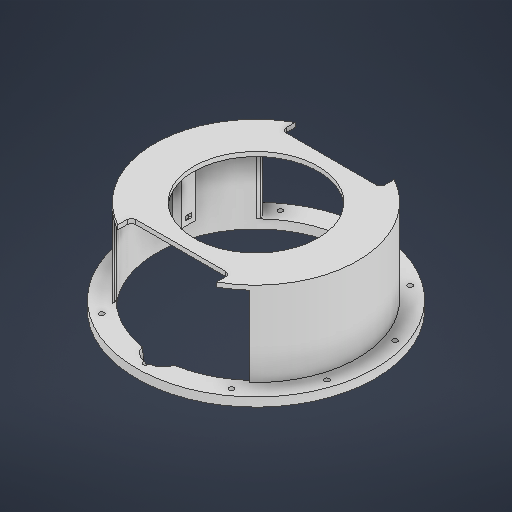
# Autodesk Inventor part: Cylinder Segment  Camera only
Saved by Autodesk Inventor 2026 (Build 300175000, 175)
## iProperties
Created: 2024-04-11
Part Number: Cylinder Segment  Camera only
Material: Generic
Document SubType Name: Modeling
Designer: Thienan Hoang
Density: 1 g/cm^3
Appearance: Default
Author: Thienan Hoang
Autodesk Inventor part; units mm, degrees
sketch "Sketch1" plane through (0, 0, 0) normal (0, 1, 0) x (-1, 0, 0)
  circle A0 centre (0, 0) radius 135
  circle A1 centre (0, 0) radius 115
  circle A2 centre (0, 0) radius 112.0375
  circle A3 centre (0, 0) radius 9.5
  circle A4 centre (0, 0) radius 125
  circle A5 centre (0, -125) radius 2.75
  circle A6 centre (73.4732, -101.1271) radius 2.75
  circle A7 centre (118.8821, -38.6271) radius 2.75
  circle A8 centre (118.8821, 38.6271) radius 2.75
  circle A9 centre (73.4732, 101.1271) radius 2.75
  circle A10 centre (0, 125) radius 2.75
  circle A11 centre (-73.4732, 101.1271) radius 2.75
  circle A12 centre (-118.8821, 38.6271) radius 2.75
  circle A13 centre (-118.8821, -38.6271) radius 2.75
  circle A14 centre (-73.4732, -101.1271) radius 2.75
  point P0 (0, -115)
  point P1 (0, -112.0375)
  point P2 (0, -135)
  point P3 (0, -112.0375)
  point P4 (0, -115)
  point P5 (0, -135)
  point P6 (0, 112.0375)
  point P7 (0, 115)
  point P8 (0, 135)
  dimension "d264" = 250
  dimension "Absolute_Diameter" = 270
  dimension "Diameter_No_Outer_Lip" = 230
  dimension "Inner_Cylinder_Diameter" = 224.075
  dimension "Lip_Diameter" = 19
  dimension "d265" = 5.5
  dimension "d268" = 360
  constraints: 14 centre point, 8 coincident, 6 point on circle, 1 vertical alignment, 23 other
  measures "Absolute_Diameter" diameter of A0
  measures "Diameter_No_Outer_Lip" diameter of A1
  measures "Inner_Cylinder_Diameter" diameter of A2
  measures "Lip_Diameter" diameter of A3
  measures "d265" diameter of A5
extrude "Extrusion1" add sketch "Sketch1" along normal blind 10 contours A0 | A4 A7 A6 A5 A14 A13 A12 A11 A10 A9 A8
extrude "Extrusion2" add sketch "Sketch1" along normal blind 105.5 contours A1
sketch "Sketch2" plane through (0, 105.5, 0) normal (0, 1, 0) x (1, 0, 0)
  circle A0 centre (0, 0) radius 115
  circle A1 centre (0, 0) radius 70.375
  dimension "Lip_Diameter_Out" = 230
  dimension "Inner_Lip_Diameter" = 140.75
  constraints: 2 centre point, 1 coincident
  measures "Lip_Diameter_Out" diameter of A0
  measures "Inner_Lip_Diameter" diameter of A1
extrude "Extrusion7" add sketch "Sketch2" against normal blind 5
sketch "Sketch28" plane through (0, 10, 0) normal (0, 1, 0) x (1, 0, 0)
  line L0 (-77.5, -75) -> (77.5, -75)
  line L1 (77.5, -75) -> (77.5, -175)
  line L2 (77.5, -175) -> (-77.5, -175)
  line L3 (-77.5, -175) -> (-77.5, -75)
  circle A0 centre (0, -125) radius 2.75 projected
  line L4 (-77.5, -75) -> (77.5, -175) construction
  line L5 (77.5, -75) -> (-77.5, -175) construction
  point P0 (0, 0)
  dimension "d271" = 155
  dimension "d272" = 100
  constraints: 12 end point, 2 midpoint, 2 parallel, 1 horizontal, 1 perpendicular
  measures "d271" distance of L1.end L2.end
  measures "d272" distance of L0.end L1.end
extrude "Extrusion34" cut sketch "Sketch28" along normal up to surface (90.5 mm away)
sketch "Sketch30" plane through (0, 10, 0) normal (0, 1, 0) x (1, 0, 0)
  point P0 (0, 0)
ref_plane "Work Plane19" through (16.25, 10, -160.125) normal (0, 0.3947439, -0.9187912) x (1, 0, 0)
ref_plane "Work Plane21" through (16.25, 10, -160.125) normal (0, 0.911762, 0.4107189) x (1, 0, 0)
ref_plane "Work Plane22" through (16.25, 101.1762, -119.0531) normal (0, 0.911762, 0.4107189) x (1, 0, 0)
sketch "Sketch31" plane through (16.25, 101.1762, -119.0531) normal (0, 0.911762, 0.4107189) x (1, 0, 0)
  circle A0 centre (-16.25, -239.1031) radius 20
  point P0 (-16.25, -150.1031)
  dimension "d286" = 40
  dimension "d289" = 89
  constraints: 1 centre point
  measures "d286" diameter of A0
  measures "d289" distance of point (-16.25, -150.103) A0.centre
extrude "Extrusion36" cut sketch "Sketch31" along normal mid plane 52.8625
fillet "Fillet19" radius 5 2 edges at (-77.5, 55.25, 80.9083) (77.5, 55.25, 80.9083)
sketch "Sketch32" plane through (0, 105.5, 0) normal (0, 1, 0) x (1, 0, 0)
  line L0 (-51, -85) -> (51, -85)
  line L1 (56, -90) -> (56, -125)
  line L2 (56, -125) -> (-56, -125)
  line L3 (-56, -125) -> (-56, -90)
  line L4 (-56, -85) -> (56, -125) construction
  line L5 (56, -85) -> (-56, -125) construction
  arc A0 (-51, -85) -> (-56, -90) centre (-51, -90) ccw
  arc A1 (56, -90) -> (51, -85) centre (51, -90) ccw
  point P0 (0, 0)
  point P1 (0, -105)
  point P2 (0, -85)
  dimension "d291" = 112
  dimension "d292" = 40
  dimension "d293" = 5
  dimension "d294" = 5
  dimension "d295" = 85
  constraints: 12 end point, 4 point on circle, 4 point on line, 4 tangent, 3 midpoint, 2 centre point, 2 parallel, 1 horizontal, 1 perpendicular
  measures "d291" distance of L1.end L2.end
  measures "d292" distance of L5.start L1.end
  measures "d293" radius of A0
  measures "d294" radius of A1
  measures "d295" distance of point (0, 0) point (0, -85)
extrude "Extrusion37" cut sketch "Sketch32" against normal blind 10
sketch "Sketch33" plane through (0, 100.5, 0) normal (0, -1, 0) x (1, 0, 0)
  circle A0 centre (0, 0) radius 70.375
  line L0 (-86.7392, 8) -> (-75, 8)
  line L1 (-75, 8) -> (-75, -8)
  line L2 (-75, -8) -> (-86.7392, -8)
  line L3 (-86.7392, -8) -> (-86.7392, 8)
  line L4 (-86.7392, 8) -> (-75, -8) construction
  line L5 (-75, 8) -> (-86.7392, -8) construction
  line L6 (0, 0) -> (0, 70.375)
  line L7 (86.7392, 8) -> (75, 8)
  line L8 (75, 8) -> (75, -8)
  line L9 (75, -8) -> (86.7392, -8)
  line L10 (86.7392, -8) -> (86.7392, 8)
  line L11 (86.7392, 8) -> (75, -8) construction
  line L12 (75, 8) -> (86.7392, -8) construction
  circle A1 centre (0, 0) radius 76.375
  point P0 (-80.8696, 0)
  point P1 (80.8696, 0)
  point P2 (-75, 0)
  point P3 (-75.9549, -8)
  point P4 (-75.9549, 8)
  point P5 (75.9549, 8)
  point P6 (75.9549, -8)
  dimension "d313" = 140.75
  dimension "d298" = 16
  dimension "d301" = 75
  dimension "d314" = 6
  constraints: 26 end point, 5 symmetric about line, 3 midpoint, 2 parallel, 1 centre point, 1 coincident, 1 horizontal, 1 perpendicular, 1 vertical, 1 vertical alignment, 2 other
  measures "d298" distance of L0.end L1.end
  measures "d301" distance of point (0, 0) point (-75, 0)
extrude "Extrusion38" add sketch "Sketch33" along normal blind 45 contours L0 A1 L2 L3 | L7 L10 L9 A1
sketch "Sketch35" plane through (0, 55.5, 0) normal (0, -1, 0) x (1, 0, 0)
  line L0 (0, 0) -> (0, 42.8625)
  arc A0 (80.604, -8) -> (-80.604, -8) centre (0, 0) ccw
  circle A1 centre (-81, 0) radius 3.5625
  circle A2 centre (81, 0) radius 3.5625
  line L1 (-82.978, -3.6069) -> (-85.1126, -0.0905)
  line L2 (-85.1126, -0.0905) -> (-83.1347, 3.5164)
  line L3 (-83.1347, 3.5164) -> (-79.022, 3.6069)
  line L4 (-79.022, 3.6069) -> (-76.8874, 0.0905)
  line L5 (-76.8874, 0.0905) -> (-78.8653, -3.5164)
  line L6 (-78.8653, -3.5164) -> (-82.978, -3.6069)
  line L7 (82.978, -3.6069) -> (85.1126, -0.0905)
  line L8 (85.1126, -0.0905) -> (83.1347, 3.5164)
  line L9 (83.1347, 3.5164) -> (79.022, 3.6069)
  line L10 (79.022, 3.6069) -> (76.8874, 0.0905)
  line L11 (76.8874, 0.0905) -> (78.8653, -3.5164)
  line L12 (78.8653, -3.5164) -> (82.978, -3.6069)
  arc A3 (75.9549, -8) -> (-75.9549, -8) centre (0, 0) ccw
  line L13 (-75.9549, -8) -> (-86.7392, -8)
  line L14 (-86.7392, -8) -> (-86.7392, 8)
  line L15 (86.7392, -8) -> (86.7392, 8)
  line L16 (-86.7392, 8) -> (-75.9549, 8) projected
  line L17 (-86.7392, 8) -> (-75.9549, 8)
  line L18 (86.7392, 8) -> (75.9549, 8)
  line L19 (-79.022, 3.6069) -> (-78.8653, -3.5164)
  line L20 (-78.8653, -3.5164) -> (-14.3502, -2.0973)
  line L21 (-14.3502, -2.0973) -> (-14.5068, 5.0259)
  line L22 (-14.5068, 5.0259) -> (-79.022, 3.6069)
  line L23 (79.022, 3.6069) -> (78.8653, -3.5164)
  line L24 (78.8653, -3.5164) -> (65.0181, -3.2118)
  line L25 (65.0181, -3.2118) -> (65.1748, 3.9115)
  line L26 (65.1748, 3.9115) -> (79.022, 3.6069)
  line L27 (86.7392, -8) -> (75.9549, -8)
  arc A4 (87.1335, -8) -> (-87.1335, -8) centre (0, 0) ccw
  point P0 (-80.9217, -3.5616)
  point P1 (-76.2966, -3.4599)
  point P2 (-76.2869, 3.667)
  point P3 (76.2869, 3.667)
  point P4 (76.2966, -3.4599)
  dimension "d309" = 7.125
  dimension "d308" = 162
  constraints: 54 end point, 10 symmetric about line, 8 point on circle, 5 equal length, 4 centre point, 4 coincident, 4 point on line, 3 perpendicular, 1 horizontal, 1 midpoint, 1 vertical, 17 other
  measures "d308" diameter of A0
extrude "Extrusion40" cut sketch "Sketch35" against normal blind 15 contours A2 L23 A0 | A0 A2 | A2 L23 | A1 L19 A0 | A0 A1 | A1 L19
extrude "Extrusion41" add sketch "Sketch35" along normal blind 5 contours L27 A3 L24 L12 A0 | A0 L12 L7 L8 L9 A2 L18 L15 L27 | L9 L26 A3 L18 A0 | L16 A3 L22 L3 A0 | A0 A1 L3 L2 L1 L6 L13 L14 L16 | L6 L20 A3 L13 A0
sketch "Sketch36" plane through (0, 50.5, 0) normal (0, -1, 0) x (1, 0, 0)
  circle A0 centre (0, 0) radius 76.375
  line L0 (-86.7392, 8) -> (-75.9549, 8) projected
  line L1 (-86.7392, -8) -> (-86.7392, 8) projected
  line L2 (-86.7392, 8) -> (-86.7392, -8)
  line L3 (-86.7392, -8) -> (-75.9549, -8)
  line L4 (-75.9549, 8) -> (-86.7392, 8)
  arc A1 (-80.9217, -3.5616) -> (-81.0783, 3.5616) centre (-81, 0) ccw projected
  circle A2 centre (-81, 0) radius 3.5667
  line L5 (0, 0) -> (0, 76.375)
  line L6 (86.7392, 8) -> (75.9549, 8)
  line L7 (86.7392, -8) -> (86.7392, 8)
  line L8 (86.7392, 8) -> (86.7392, -8)
  line L9 (86.7392, -8) -> (75.9549, -8)
  line L10 (75.9549, 8) -> (86.7392, 8)
  arc A3 (81.0783, 3.5616) -> (80.9217, -3.5616) centre (81, 0) ccw
  circle A4 centre (81, 0) radius 3.5667
  constraints: 18 end point, 9 symmetric about line, 4 centre point, 3 coincident, 3 point on circle, 2 equal length, 1 perpendicular, 1 vertical, 2 other
extrude "Extrusion42" add sketch "Sketch36" along normal blind 5 contours A0 L6 L7 L9 | L3 L1 L0 A0
ref_plane "Work Plane25" through (0, 0, 0) normal (0, 0, 1) x (1, 0, 0)
ref_plane "Work Plane23" through (0, 0, 135) normal (0, 0, 1) x (1, 0, 0)
ref_plane "Work Plane24" through (0, 0, -135) normal (0, 0, -1) x (-1, 0, 0)
mirror "Mirror1" about plane through (0, 0, 0) normal (0, 0, 1) of "Extrusion34", "Extrusion36", "Fillet19", "Extrusion37", "Extrusion38", "Extrusion40", "Extrusion41", "Extrusion42"
ref_plane "Work Plane26" through (16.25, 10, 160.125) normal (0, -0.3947439, -0.9187912) x (1, 0, 0)
ref_plane "Work Plane27" through (16.25, 10, 160.125) normal (0, -0.911762, 0.4107189) x (1, 0, 0)
ref_plane "Work Plane28" through (16.25, 101.1762, 119.0531) normal (0, -0.911762, 0.4107189) x (1, 0, 0)
body "Solid1"
